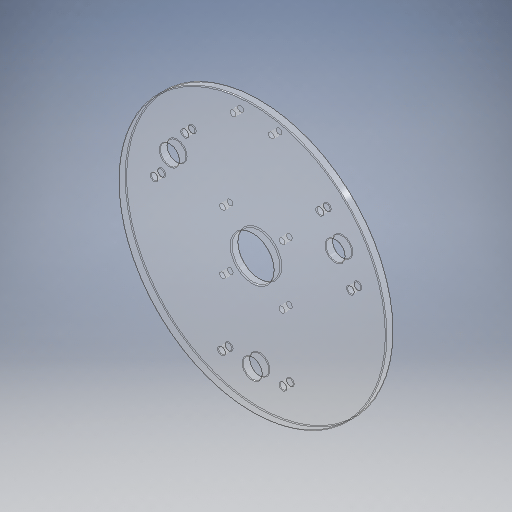
# Autodesk Inventor part: Topo
Saved by Autodesk Inventor 2025.1 (Build 291241020, 241B)
## iProperties
Created: 2025-05-02
Part Number: Topo
Material: Generic
Document SubType Name: Modeling
Designer: Nelson
Density: 1 g/cm^3
Appearance: Polycarbonate - Clear
Author: Nelson
Autodesk Inventor part; units mm, degrees
ref_plane "YZ Plane" through (0, 0, 0) normal (1, 0, 0) x (0, 1, 0)
ref_plane "XZ Plane" through (0, 0, 0) normal (0, 1, 0) x (-1, 0, 0)
ref_plane "XY Plane" through (0, 0, 0) normal (0, 0, 1) x (1, 0, 0)
sketch "Sketch1" plane through (0, 0, 0) normal (0, 0, 1) x (1, 0, 0)
  circle A0 centre (0, 0) radius 70
  circle A1 centre (0, 0) radius 50 construction
  circle A2 centre (0, -50) radius 5
  line L0 (0, -50) -> (16, -50) construction
  circle A3 centre (16, -50) radius 1.75
  line L1 (0, -50) -> (-16, -50) construction
  circle A4 centre (-16, -50) radius 1.75
  circle A5 centre (35.3013, 38.8564) radius 1.75
  line L2 (43.3013, 25) -> (35.3013, 38.8564) construction
  circle A6 centre (43.3013, 25) radius 5
  line L3 (43.3013, 25) -> (51.3013, 11.1436) construction
  circle A7 centre (51.3013, 11.1436) radius 1.75
  circle A8 centre (-51.3013, 11.1436) radius 1.75
  line L4 (-43.3013, 25) -> (-51.3013, 11.1436) construction
  circle A9 centre (-43.3013, 25) radius 5
  line L5 (-43.3013, 25) -> (-35.3013, 38.8564) construction
  circle A10 centre (-35.3013, 38.8564) radius 1.75
  circle A11 centre (0, 0) radius 11
  line L6 (0, 0) -> (0, 60.58) construction
  line L7 (0, 60.58) -> (0, 45.08)
  line L8 (0, 60.58) -> (10.001, 60.58) construction
  line L9 (0, 60.58) -> (-10.001, 60.58) construction
  circle A12 centre (10.001, 60.58) radius 1.5
  circle A13 centre (-10.001, 60.58) radius 1.5
  line L10 (-15.5, 0) -> (15.5, 0) construction
  line L11 (0, -15.5) -> (0, 15.5) construction
  circle A14 centre (15.5, 15.5) radius 1.5
  circle A15 centre (-15.5, 15.5) radius 1.5
  circle A16 centre (15.5, -15.5) radius 1.5
  circle A17 centre (-15.5, -15.5) radius 1.5
  dimension "D_F" = 100
  dimension "D_B" = 140
  dimension "Furos" = 10
  dimension "d3" = 16
  dimension "d4" = 3.5
  dimension "d5" = 16
  dimension "d6" = 3.5
  dimension "d9" = 360
  dimension "d11" = 22
  dimension "d17" = 60.58
  dimension "d18" = 15.5
  dimension "d19" = 10.001
  dimension "d23" = 10.001
  dimension "d24" = 3
  dimension "d25" = 3
  dimension "d26" = 31
  dimension "d27" = 31
  dimension "FN" = 3
  dimension "d29" = 15.5
  dimension "d30" = 15.5
  constraints: 24 end point, 17 centre point, 11 coincident, 5 horizontal, 5 point on line, 3 symmetric about line, 2 midpoint, 1 vertical, 1 vertical alignment, 36 other
  measures "D_B" diameter of A0
  measures "Furos" diameter of A2
  measures "d3" distance of L0.start L0.end
  measures "d4" diameter of A3
  measures "d5" distance of L0.start L1.end
  measures "d6" diameter of A4
  measures "d11" diameter of A11
  measures "d17" distance of L6.start L6.end
  measures "d18" distance of L6.end L7.end
  measures "d19" distance of L6.end L8.end
  measures "d23" distance of L6.end L9.end
  measures "d24" diameter of A12
  measures "d25" diameter of A13
  measures "d26" distance of L10.start L10.end
  measures "d27" distance of L11.start L11.end
  measures "FN" diameter of A14
  measures "d29" distance of L10.end A14.centre
  measures "d30" distance of L11.end A14.centre
extrude "Extrusion1" add sketch "Sketch1" along normal blind 4
fillet "Fillet1" radius 0.4 2 edges at (-70, 0, 4) (-70, 0, 0)
fillet "Fillet2" radius 0.5 2 edges at (-11, 0, 0) (-11, 0, 4)
fillet "Fillet3" radius 0.3 18 edges at (33.5513, 38.8564, 4) (38.3013, 25, 4) (49.5513, 11.1436, 4) (14.25, -50, 4) (-5, -50, 4) (-17.75, -50, 4) (-53.0513, 11.1436, 4) (-48.3013, 25, 4) (-37.0513, 38.8564, 4) (-17.75, -50, 0) (-5, -50, 0) (14.25, -50, 0) (49.5513, 11.1436, 0) (38.3013, 25, 0) (33.5513, 38.8564, 0) (-37.0513, 38.8564, 0) (-48.3013, 25, 0) (-53.0513, 11.1436, 0)
body "Solid1"
